Window Frame_v2 (Autodesk Fusion 360 design; units mm, degrees)
Autodesk Fusion 360 part; units mm, degrees
sketch "Sketch1" plane through (0, 0, 0) normal (0, 1, 0) x (1, 0, 0)
  line L0 (-12.55, -12.55) -> (12.55, -12.55)
  line L1 (12.55, -12.55) -> (12.55, 12.55)
  line L2 (12.55, 12.55) -> (-12.55, 12.55)
  line L3 (-12.55, 12.55) -> (-12.55, -12.55)
  line L4 (-12.55, -12.55) -> (12.55, 12.55) construction
  line L5 (12.55, -12.55) -> (-12.55, 12.55) construction
  line L6 (-10.5, -10.5) -> (10.5, -10.5)
  line L7 (10.5, -10.5) -> (10.5, 10.5)
  line L8 (10.5, 10.5) -> (-10.5, 10.5)
  line L9 (-10.5, 10.5) -> (-10.5, -10.5)
  line L10 (-10.5, -10.5) -> (10.5, 10.5) construction
  line L11 (10.5, -10.5) -> (-10.5, 10.5) construction
  dimension "d1" = 25.1
  dimension "d2" = 25.1
  dimension "d3" = 21
  dimension "d4" = 21
  constraint horizontal L0
  constraint perpendicular L0 L1
  constraint parallel L0 L2
  constraint parallel L1 L3
  constraint coincident L4 origin
  constraint coincident L5 origin
  constraint horizontal L6
  constraint perpendicular L6 L7
  constraint parallel L6 L8
  constraint parallel L7 L9
  constraint coincident L10 origin
  constraint coincident L11 origin
  measures "d1" distance of L1.end L2.end
  measures "d2" distance of L0.end L1.end
  measures "d3" distance of L7.end L8.end
  measures "d4" distance of L6.end L7.end
extrude "Extrude1" add sketch "Sketch1" along normal blind 2
chamfer "Chamfer1" distance 2 angle 45 4 edges at (-10.5, 0, 0) (0, 0, 10.5) (10.5, 0, 0) (0, 0, -10.5) measured on face at (-10.5, 0.6667, -3.5) measured on face at (-3.5, 0.6667, 10.5) measured on face at (10.5, 0.6667, 3.5) measured on face at (3.5, 0.6667, -10.5)
